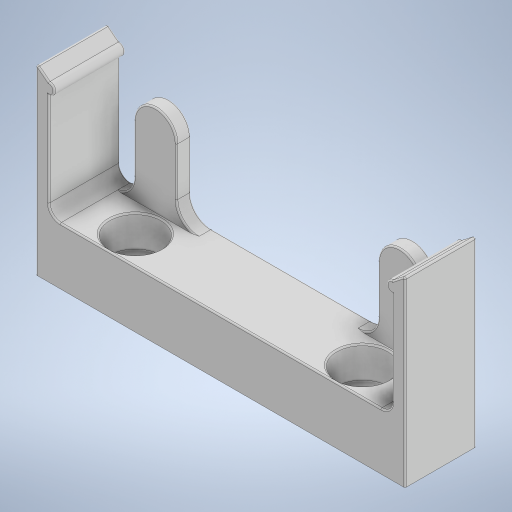
# Autodesk Inventor part: Top bot holder
Saved by Autodesk Inventor 2024 (Build 280153000, 153)
## iProperties
Created: 2024-04-04
Part Number: Top bot holder
Material: Generic
Document SubType Name: Modeling
Designer: jens1
Density: 1 g/cm^3
Appearance: Default
Author: jens1
## iProperties of the stored document Top bot holder_3DPrint.ipt
Created: 2024-04-04
Part Number: Top bot holder_3DPrint
Material: Generic
Document SubType Name: Modeling
Designer: jens1
Density: 1 g/cm^3
Appearance: Default
Author: jens1
Autodesk Inventor part; units mm, degrees
ref_plane "YZ Plane" through (0, 0, 0) normal (1, 0, 0) x (0, 1, 0)
ref_plane "XZ Plane" through (0, 0, 0) normal (0, 1, 0) x (-1, 0, 0)
ref_plane "XY Plane" through (0, 0, 0) normal (0, 0, 1) x (1, 0, 0)
sketch "Sketch1" plane through (0, 0, 0) normal (0, 0, 1) x (1, 0, 0)
  line L0 (0, 0) -> (65, 0)
  line L1 (65, 0) -> (65, 10)
  line L2 (65, 10) -> (0, 10)
  line L3 (0, 10) -> (0, 0)
  line L4 (0, 10) -> (2.25, 10)
  line L5 (2.25, 10) -> (2.25, 30.5)
  line L6 (2.25, 30.5) -> (0, 30.5)
  line L7 (0, 30.5) -> (0, 10)
  circle A0 centre (2.25, 29.5) radius 1
  line L8 (65, 10) -> (62.75, 10)
  line L9 (62.75, 10) -> (62.75, 30.5)
  line L10 (62.75, 30.5) -> (65, 30.5)
  line L11 (65, 30.5) -> (65, 10)
  circle A1 centre (62.75, 29.5) radius 1
  line L12 (65, 30.5) -> (62.75, 30.5)
  line L13 (62.75, 30.5) -> (62.75, 32.25)
  line L14 (62.75, 32.25) -> (65, 32.25)
  line L15 (65, 32.25) -> (65, 30.5)
  line L16 (65, 32.25) -> (62.75, 30.5)
  line L17 (2.25, 30.5) -> (0, 30.5)
  line L18 (0, 30.5) -> (0, 32.25)
  line L19 (0, 32.25) -> (2.25, 32.25)
  line L20 (2.25, 32.25) -> (2.25, 30.5)
  line L21 (0, 32.25) -> (2.25, 30.5)
  point P0 (62.75, 28.5)
  point P1 (2.25, 10)
  point P2 (2.25, 28.5)
  dimension "d4" = 2
  dimension "d7" = 2
  dimension "d0" = 65
  dimension "d1" = 10
  dimension "d2" = 2.25
  dimension "d3" = 20.5
  dimension "d5" = 2.25
  dimension "d6" = 20.5
  dimension "d42" = 2.25
  dimension "d43" = 1.75
  dimension "d44" = 2.25
  dimension "d45" = 1.75
  constraints: 44 end point, 10 parallel, 5 horizontal, 5 perpendicular, 2 point on line, 6 other
  measures "d0" distance of L2.end L1.end
  measures "d1" distance of L1.end L0.end
  measures "d2" distance of L6.end L5.end
  measures "d3" distance of L5.end L4.end
  measures "d5" distance of L9.end L10.end
  measures "d6" distance of L8.end L9.end
  measures "d42" distance of L13.end L14.end
  measures "d43" distance of L12.end L13.end
  measures "d44" distance of L18.end L19.end
  measures "d45" distance of L17.end L18.end
extrude "Extrusion1" add sketch "Sketch1" along normal blind 10 contours L3 L2 L1 L0 | L7 L6 A0 L5 L2 | L2 L9 A1 L10 L11 | L18 L21 L6 | L10 L16 L15 | A0 L5 | L5 A0 | A1 L9 | L9 A1
fillet "Fillet1" radius 2 2 edges at (2.25, 10, 5) (62.75, 10, 5)
fillet "Fillet2" radius 0.25 2 edges at (0, 32.25, 5) (65, 32.25, 5)
sketch "Sketch2" plane through (4.25, 10, 0) normal (0, 1, 0) x (1, 0, 0)
  line L0 (-4.25, 0) -> (60.75, 0) projected
  line L1 (60.75, 0) -> (60.75, -10) projected
  line L2 (-4.25, -10) -> (60.75, -10) projected
  line L3 (-4.25, 0) -> (-4.25, -10) projected
  point P0 (8.25, -5)
  point P1 (48.25, -5)
  dimension "d12" = 0
  dimension "d13" = 40
  dimension "d14" = 12.5
  dimension "d15" = 5
  measures "d12" vertical distance of point (48.25, -5) point (8.25, -5)
  measures "d13" distance of point (8.25, -5) point (48.25, -5)
  measures "d14" distance from line of L3 point (8.25, -5)
  measures "d15" distance from line of L0 point (48.25, -5)
hole "Hole1" at (12.5, 10, 5) at (52.5, 10, 5) direction (0, -1, 0) diameter 5.5 end through all counterbore diameter 9 counterbore depth 5.5
chamfer "Chamfer1" distance 0.25 angle 45 2 edges at (12.5, 10, 0.5) (52.5, 10, 0.5)
chamfer "Chamfer2" distance 0.25 angle 45 2 edges at (12.5, 4.5, 2.25) (52.5, 4.5, 2.25)
sketch "Sketch3" plane through (0, 0, 0) normal (0, 0, -1) x (-1, 0, 0)
  line L0 (0, 0) -> (0, 29.5) projected
  arc A0 (0, 29.5) -> (-1, 30.5) centre (-1, 29.5) ccw projected
  line L1 (-1, 30.5) -> (-2.25, 30.5) projected
  line L2 (-2.25, 28.5) -> (-2.25, 12) projected
  arc A1 (-2.25, 30.5) -> (-2.25, 28.5) centre (-2.25, 29.5) ccw projected
  arc A2 (-4.25, 10) -> (-2.25, 12) centre (-4.25, 12) ccw projected
  line L3 (-4.25, 10) -> (-17.25, 10) projected
  line L4 (-17.25, 10) -> (-57.25, 10) projected
  line L5 (-57.25, 10) -> (-60.75, 10) projected
  arc A3 (-62.75, 12) -> (-60.75, 10) centre (-60.75, 12) ccw projected
  line L6 (-62.75, 12) -> (-62.75, 28.5) projected
  arc A4 (-62.75, 28.5) -> (-62.75, 30.5) centre (-62.75, 29.5) ccw projected
  line L7 (-62.75, 30.5) -> (-64, 30.5) projected
  arc A5 (-64, 30.5) -> (-65, 29.5) centre (-64, 29.5) ccw projected
  line L8 (-65, 29.5) -> (-65, 0) projected
  line L9 (-65, 0) -> (0, 0) projected
  arc A6 (-64.5965, 31.9362) -> (-65, 31.7388) centre (-64.75, 31.7388) ccw projected
  line L10 (-65, 0) -> (-65, 31.7388) projected
  line L11 (0, 0) -> (-65, 0) projected
  line L12 (0, 31.7388) -> (0, 0) projected
  arc A7 (0, 31.7388) -> (-0.4035, 31.9362) centre (-0.25, 31.7388) ccw projected
  line L13 (-2.25, 30.5) -> (-0.4035, 31.9362) projected
  arc A8 (-2.25, 30.5) -> (-2.25, 28.5) centre (-2.25, 29.5) ccw projected
  line L14 (-2.25, 12) -> (-2.25, 28.5) projected
  arc A9 (-4.25, 10) -> (-2.25, 12) centre (-4.25, 12) ccw projected
  line L15 (-60.75, 10) -> (-4.25, 10) projected
  arc A10 (-62.75, 12) -> (-60.75, 10) centre (-60.75, 12) ccw projected
  line L16 (-62.75, 28.5) -> (-62.75, 12) projected
  arc A11 (-62.75, 28.5) -> (-62.75, 30.5) centre (-62.75, 29.5) ccw projected
  line L17 (-64.5965, 31.9362) -> (-62.75, 30.5) projected
  point P0 (-62.75, 30.5)
extrude "Extrusion2" add sketch "Sketch3" against normal blind 0.25
sketch "Sketch4" plane through (0, 0, 0) normal (0, 0, -1) x (-1, 0, 0)
  arc A0 (-4.25, 10) -> (-2.25, 12) centre (-4.25, 12) ccw projected
  arc A1 (-62.75, 12) -> (-60.75, 10) centre (-60.75, 12) ccw projected
  line L0 (-57.75, 10) -> (-50.25, 10)
  line L1 (-50.25, 10) -> (-50.25, 26)
  line L2 (-50.25, 26) -> (-57.75, 26)
  line L3 (-57.75, 26) -> (-57.75, 10)
  line L4 (-14.75, 10) -> (-7.25, 10)
  line L5 (-7.25, 10) -> (-7.25, 26)
  line L6 (-7.25, 26) -> (-14.75, 26)
  line L7 (-14.75, 26) -> (-14.75, 10)
  line L8 (-65, 0) -> (-65, 31.7388) projected
  line L9 (0, 0) -> (-65, 0) projected
  line L10 (0, 31.7388) -> (0, 0) projected
  arc A2 (0, 31.7388) -> (-0.4035, 31.9362) centre (-0.25, 31.7388) ccw projected
  line L11 (-2.25, 30.5) -> (-0.4035, 31.9362) projected
  arc A3 (-2.25, 30.5) -> (-2.25, 28.5) centre (-2.25, 29.5) ccw projected
  line L12 (-2.25, 12) -> (-2.25, 28.5) projected
  line L13 (-60.75, 10) -> (-4.25, 10) projected
  line L14 (-62.75, 28.5) -> (-62.75, 12) projected
  arc A4 (-62.75, 28.5) -> (-62.75, 30.5) centre (-62.75, 29.5) ccw projected
  line L15 (-64.5965, 31.9362) -> (-62.75, 30.5) projected
  arc A5 (-64.5965, 31.9362) -> (-65, 31.7388) centre (-64.75, 31.7388) ccw projected
  dimension "d36" = 7.5
  constraints: 16 end point, 4 parallel, 2 horizontal, 2 perpendicular, 1 collinear, 1 point on line
  measures "d36" distance between parallel lines of L1 L3
extrude "Extrusion3" add sketch "Sketch4" along normal blind 2.5
fillet "Fillet5" radius 3.75 4 edges at (7.25, 26, -1.25) (14.75, 26, -1.25) (50.25, 26, -1.25) (57.75, 26, -1.25)
fillet "Fillet6" radius 3.75 4 edges at (57.75, 10, -1.25) (50.25, 10, -1.25) (7.25, 10, -1.25) (14.75, 10, -1.25)
fillet "Fillet7" radius 0.25 39 edges at (50.25, 18, -2.5) (51.3483, 24.9017, -2.5) (54, 26, -2.5) (56.6517, 24.9017, -2.5) (57.75, 17.9622, -2.5) (14.75, 18.0001, -2.5) (11, 26, -2.5) (8.3483, 24.9017, -2.5) (13.6517, 24.9017, -2.5) (7.25, 17.9622, -2.5) (2.8358, 10.5858, -2.5) (62.1642, 10.5858, -2.5) (56.6517, 24.9017, 0) (54, 26, 0) (51.3483, 24.9017, 0) (57.75, 17.9622, 0) (50.25, 18, 0) (14.75, 18.0001, 0) (7.25, 17.9622, 0) (11, 26, 0) (8.3483, 24.9017, 0) (13.6517, 24.9017, 0) (0, 15.8694, 10) (65, 15.8694, 10) (0.1402, 31.9634, -2.5) (1.3267, 31.2181, -2.5) (0, 15.8694, -2.5) (3.25, 29.5, -2.5) (64.8598, 31.9634, -2.5) (63.6733, 31.2181, -2.5) (65, 15.8694, -2.5) (61.75, 29.5, -2.5) (2.8358, 10.5858, 10) (2.25, 20.25, 10) (62.1642, 10.5858, 10) (62.75, 20.25, 10) (32.5, 10, 10) (3.25, 29.5, 10) (61.75, 29.5, 10)
equation "\"d2\" = d5"
equation "\"d45\" = d43"
body "Solid1"
